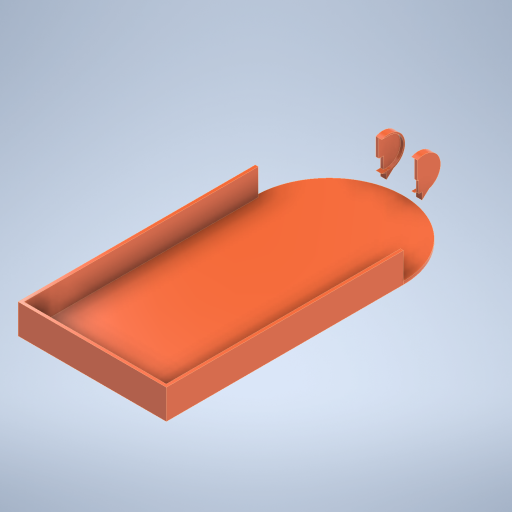
# Autodesk Inventor part: korpus
Saved by Autodesk Inventor 2024 (Build 280153000, 153)
## iProperties
Created: 2025-05-20
Part Number: korpus
Material: Ogólny
Document SubType Name: Modeling
Designer: Paweł
Density: 1 g/cm^3
Appearance: Gładki — jasnopomarańczowy
Author: Paweł
Autodesk Inventor part; units mm, degrees
ref_plane "YZ Plane" through (0, 0, 0) normal (1, 0, 0) x (0, 1, 0)
ref_plane "XZ Plane" through (0, 0, 0) normal (0, 1, 0) x (-1, 0, 0)
ref_plane "XY Plane" through (0, 0, 0) normal (0, 0, 1) x (1, 0, 0)
sketch "Szkic1" plane through (0, 0, 0) normal (0, 1, 0) x (-1, 0, 0)
  line L0 (125, 200) -> (-125, 200)
  line L1 (-125, 200) -> (-125, -200)
  line L2 (-125, -200) -> (125, -200)
  line L3 (125, -200) -> (125, 200)
  arc A0 (-125, -200) -> (125, -200) centre (0, -200) ccw
  arc A1 (-115, -200) -> (115, -200) centre (0, -200) ccw
  line L4 (115, -200) -> (115, 190)
  line L5 (115, 190) -> (-115, 190)
  line L6 (-115, 190) -> (-115, -200)
  point P0 (0, 0)
  point P1 (0, 200)
  point P2 (125, 0)
  dimension "d0" = 400
  dimension "d1" = 250
  dimension "d4" = 10
  dimension "d5" = 10
  constraints: 14 end point, 4 point on circle, 3 midpoint, 3 parallel, 2 centre point, 2 perpendicular, 1 coincident, 1 horizontal, 1 horizontal alignment, 1 tangent, 1 vertical alignment, 2 other
  measures "d0" distance of L2.end L0.start
  measures "d1" distance of L0.start L0.end
  measures "d4" radial gap between concentric circles of A0 A1
  measures "d5" distance between parallel lines of L3 L4
extrude "Wyciągnięcie proste1" add sketch "Szkic1" along normal blind 5
sketch "Szkic2" plane through (0, 5, 0) normal (0, 1, 0) x (1, 0, 0)
  line L0 (125, -200) -> (125, 200) projected
  arc A0 (125, 200) -> (-125, 200) centre (0, 200) ccw projected
  line L1 (-125, 200) -> (-125, -200) projected
  line L2 (-125, -200) -> (125, -200) projected
  line L3 (-120, -195) -> (-120, 200)
  arc A1 (120, 200) -> (-120, 200) centre (0, 200) ccw
  line L4 (120, 200) -> (120, -195)
  line L5 (120, -195) -> (-120, -195)
  line L6 (-125, -200) -> (125, -200)
  line L7 (125, -200) -> (125, 200)
  line L8 (125, 200) -> (-125, 200)
  line L9 (-125, 200) -> (-125, -200)
  point P0 (0, 0)
  point P1 (120, 200)
  dimension "d6" = 5
  constraints: 14 end point, 2 parallel, 2 point on circle, 1 centre point, 1 horizontal, 1 perpendicular, 3 other
  measures "d6" distance between parallel lines of L1 L3
extrude "Wyciągnięcie proste2" add sketch "Szkic2" along normal blind 45 contours L2 L1 L8 L3 L5 L4 L0
sketch "Szkic11" plane through (0, 0, 0) normal (1, 0, 0) x (0, 1, 0)
  circle A0 centre (55, -325) radius 25
  circle A1 centre (55, -325) radius 27.5
  line L0 (30, -325) -> (27.5, -325)
  line L1 (80, -325) -> (82.5, -325)
  line L2 (30, -325) -> (30, -313.5436)
  line L3 (80, -325) -> (80, -313.5436)
  line L4 (5, -325) -> (5, -200) projected
  point P0 (0, 0)
  dimension "d27" = 50
  dimension "d28" = 55
  dimension "d29" = 25
  constraints: 8 end point, 6 point on circle, 2 centre point, 2 horizontal, 2 vertical, 1 coincident, 1 horizontal alignment
  measures "d27" diameter of A0
  measures "d28" diameter of A1
  measures "d29" distance from line of L4 L0.start
extrude "Wyciągnięcie proste8" add sketch "Szkic11" along normal mid plane 60 contours L1 A1 L0 A0 | L3 A1 L1 | L0 A1 L2
sketch "Szkic12" plane through (0, 0, 0) normal (1, 0, 0) x (0, 1, 0)
  point P0 (0, 0)
sketch "Szkic13" plane through (0, 0, 0) normal (1, 0, 0) x (0, 1, 0)
  line L0 (30, -325) -> (30, -313.5436) projected
  arc A0 (30, -313.5436) -> (80, -313.5436) centre (55, -325) ccw projected
  line L1 (80, -313.5436) -> (80, -325) projected
  arc A1 (30, -325) -> (80, -325) centre (55, -325) ccw projected
  point P0 (0, 0)
extrude "Wyciągnięcie proste9" cut sketch "Szkic13" along normal mid plane 50
sketch "Szkic17" plane through (-30, 0, 0) normal (-1, 0, 0) x (0, 0, 1)
  line L0 (-321.3466, 27.7438) -> (-321.3466, 30) projected
  line L1 (-321.3466, 27.7438) -> (-321.3466, 17.7438)
  arc A0 (-313.5436, 80) -> (-313.5436, 30) centre (-325, 55) ccw projected
  line L2 (-321.3466, 17.7438) -> (-333.5774, 28.8719)
  line L3 (-313.5436, 30) -> (-325, 30) projected
  line L4 (-313.5436, 30) -> (-313.5436, 80)
  arc A1 (-325, 80) -> (-325, 30) centre (-325, 55) ccw projected
  line L5 (-325, 80) -> (-313.5436, 80) projected
  point P0 (0, 0)
  dimension "d40" = 10
  constraints: 6 end point, 1 perpendicular, 1 point on circle, 1 vertical
  measures "d40" distance of L0.start L1.end
extrude "Wyciągnięcie proste12" add sketch "Szkic17" against normal blind 5 contours L1 L2 A0
sketch "Szkic18" plane through (30, 0, 0) normal (1, 0, 0) x (0, 0, -1)
  line L0 (313.5436, 30) -> (325, 30) projected
  arc A0 (325, 30) -> (325, 80) centre (325, 55) ccw projected
  line L1 (325, 80) -> (313.5436, 80) projected
  arc A1 (333.5774, 28.8719) -> (313.5436, 80) centre (325, 55) ccw projected
  line L2 (333.5774, 28.8719) -> (321.3466, 17.7438) projected
  line L3 (321.3466, 17.7438) -> (321.3466, 27.7438) projected
  arc A2 (313.5436, 30) -> (321.3466, 27.7438) centre (325, 55) ccw projected
  point P0 (0, 0)
extrude "Wyciągnięcie proste13" add sketch "Szkic18" against normal blind 5
sketch "Szkic19" plane through (-30, 0, 0) normal (-1, 0, 0) x (0, 0, 1)
  arc A0 (-313.5436, 80) -> (-333.5774, 28.8719) centre (-325, 55) ccw projected
  line L0 (-313.5436, 30) -> (-325, 30) projected
  arc A1 (-325, 80) -> (-325, 30) centre (-325, 55) ccw projected
  line L1 (-325, 80) -> (-313.5436, 80) projected
  arc A2 (-313.5436, 80) -> (-333.5774, 28.8719) centre (-325, 55) ccw projected
  line L2 (-333.5774, 28.8719) -> (-321.3466, 17.7438) projected
  line L3 (-313.5436, 80) -> (-313.5436, 50)
  line L4 (-200, 50) -> (-321.3466, 50) projected
  line L5 (-321.3466, 30) -> (-321.3466, 50) projected
  line L6 (-321.3466, 50) -> (-321.3466, 30)
  line L7 (-321.3466, 17.7438) -> (-321.3466, 27.7438) projected
  arc A3 (-321.3466, 27.7438) -> (-313.5436, 30) centre (-325, 55) ccw projected
  point P0 (0, 0)
  constraints: 4 end point, 1 perpendicular, 1 point on line, 1 vertical
extrude "Wyciągnięcie proste14" add sketch "Szkic19" along normal blind 5
sketch "Szkic21" plane through (30, 0, 0) normal (1, 0, 0) x (0, 0, -1)
  line L0 (321.3466, 30) -> (316.1895, 30) projected
  line L1 (321.3466, 30) -> (321.3466, 50) projected
  line L2 (321.3466, 30) -> (325, 30) projected
  arc A0 (325, 30) -> (325, 80) centre (325, 55) ccw projected
  line L3 (325, 80) -> (313.5436, 80) projected
  line L4 (313.5436, 50) -> (313.5436, 80) projected
  line L5 (316.1895, 50) -> (313.5436, 50) projected
  line L6 (316.1895, 30) -> (316.1895, 50) projected
  arc A1 (333.5774, 28.8719) -> (313.5436, 80) centre (325, 55) ccw projected
  line L7 (333.5774, 28.8719) -> (321.3466, 17.7438) projected
  line L8 (321.3466, 17.7438) -> (321.3466, 50) projected
  point P0 (0, 0)
extrude "Wyciągnięcie proste15" add sketch "Szkic21" along normal blind 5
